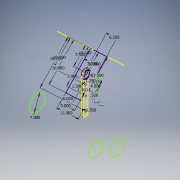
# Autodesk Inventor part: RollerIntakePrototype 2.0 3 WHEELS
Saved by Autodesk Inventor 2018.3 (Build 223284000, 284)
## iProperties
Created: 2020-01-29
Part Number: RollerIntakePrototype 2.0 3 WHEELS
Material: Generic
Document SubType Name: Modeling
Designer: 22oktynich
Density: 1 g/cm^3
Appearance: Default
Author: 22oktynich
Autodesk Inventor part; units mm, degrees
ref_plane "YZ Plane" through (0, 0, 0) normal (1, 0, 0) x (0, 1, 0)
ref_plane "XZ Plane" through (0, 0, 0) normal (0, 1, 0) x (-1, 0, 0)
ref_plane "XY Plane" through (0, 0, 0) normal (0, 0, 1) x (1, 0, 0)
sketch "Sketch1" plane through (0, 0, 0) normal (0, 0, 1) x (1, 0, 0)
  line L0 (0, 0) -> (-254, 0)
  line L1 (-254, 406.4) -> (0, 406.4)
  line L2 (0, 406.4) -> (0, 0)
  line L3 (-254, 0) -> (-254, 155.9052)
  line L4 (-285.75, 187.6552) -> (-355.6, 187.6552)
  circle A0 centre (-95.25, 190.5) radius 38.1
  arc A1 (-254, 155.9052) -> (-285.75, 187.6552) centre (-285.75, 155.9052) ccw
  circle A2 centre (-330.2, 463.55) radius 19.05
  line L5 (-515.6961, 0) -> (516.0768, 0) projected
  line L6 (-368.3, 304.8) -> (-355.6, 187.6552)
  circle A3 centre (-228.6, 355.6) radius 19.05
  circle A4 centre (279.7806, 579.9282) radius 88.9
  circle A5 centre (-152.4, 276.86) radius 19.05
  line L7 (-336.55, 187.6552) -> (-368.3, 304.8)
  point P0 (-254, 187.6552)
  dimension "d0" = 406.4
  dimension "d4" = 158.75
  dimension "d5" = 190.5
  dimension "d6" = 76.2
  dimension "d13" = 31.75
  dimension "d14" = 463.55
  dimension "d20" = 330.2
  dimension "d54" = 101.6
  dimension "d59" = 254
  dimension "d61" = 304.8
  dimension "d62" = 187.6552
  dimension "d63" = 12.7
  dimension "d76" = 38.1
  dimension "d87" = 228.6
  dimension "d88" = 355.6
  dimension "d89" = 38.1
  dimension "d90" = 177.8
  dimension "d91" = 38.1
  dimension "d92" = 276.86
  dimension "d93" = 152.4
  dimension "d94" = 82.55
  constraints: 14 end point, 6 centre point, 4 point on line, 2 point on circle, 2 tangent, 1 horizontal, 1 parallel, 1 vertical
  measures "d0" distance between parallel lines of L1 L0
  measures "d4" distance from line of L3 A0.centre
  measures "d5" distance from line of L0 A0.centre
  measures "d6" diameter of A0
  measures "d13" radius of A1
  measures "d14" distance from line of L0 A2.centre
  measures "d20" distance from line of L2 A2.centre
  measures "d54" distance from line of L4.end L3
  measures "d59" distance between parallel lines of L3 L2
  measures "d61" distance from line of L5 L6.start
  measures "d62" distance from line of L5 L4.end
  measures "d63" horizontal distance of L6.start L4.end
  measures "d76" diameter of A3
  measures "d87" distance from line of L2 A3.centre
  measures "d88" distance from line of L0 A3.centre
  measures "d89" diameter of A2
  measures "d90" diameter of A4
  measures "d91" diameter of A5
  measures "d92" distance from line of L5 A5.centre
  measures "d93" distance from line of L2 A5.centre
  measures "d94" distance from line of L3 L7.start
sketch "Sketch5" plane through (0, 0, 0) normal (0, 0, 1) x (1, 0, 0)
  line L0 (-346.559, 517.9919) -> (-91.3724, 246.8562)
  line L1 (-91.3724, 246.8562) -> (-49.3064, 146.7099)
  line L2 (-49.3064, 146.7099) -> (-96.1423, 127.0367)
  line L3 (-96.1423, 127.0367) -> (-134.6544, 218.7223)
  line L4 (-134.6544, 218.7223) -> (-383.5128, 483.1343)
  line L5 (-383.5128, 483.1343) -> (-346.5202, 517.9508)
  point P0 (0, 0)
  point P1 (-95.25, 190.5)
  point P2 (-152.4, 276.86)
  point P3 (-228.6, 355.6)
  point P4 (-330.2, 463.55)
  dimension "d107" = 50.8
  dimension "d108" = 50.8
  dimension "d109" = 25.4
  dimension "d110" = 25.4
  dimension "d111" = 25.4
  dimension "d113" = 50.8
  constraints: 12 end point, 3 perpendicular, 1 parallel, 1 point on line
  measures "d107" distance of L4.end L5.end
  measures "d108" distance from line of point (-330.2, 463.55) L5
  measures "d109" distance from line of L0 point (-330.2, 463.55)
  measures "d110" distance from line of L0 point (-228.6, 355.6)
  measures "d111" distance from line of L1 point (-95.25, 190.5)
  measures "d113" distance of L1.end L2.end
extrude "Extrusion4" add sketch "Sketch5" along normal blind 25.4
hole "Hole1" at (-95.25, 190.5, 0) at (-152.4, 276.86, 0) at (-228.6, 355.6, 0) at (-330.2, 463.55, 0) direction (0, 0, 1) diameter 22.225 end through all
sketch "Sketch6" plane through (0, 0, 25.4) normal (0, 0, 1) x (1, 0, 0)
  line L0 (-108.2166, 155.7818) -> (-61.3806, 175.455)
  line L1 (-49.3064, 146.7099) -> (-91.3724, 246.8562) projected
  line L2 (-61.3806, 175.455) -> (-49.3064, 146.7099)
  line L3 (-134.6544, 218.7223) -> (-96.1423, 127.0367) projected
  line L4 (-49.3064, 146.7099) -> (-96.1423, 127.0367)
  line L5 (-96.1423, 127.0367) -> (-108.2166, 155.7818)
  circle A0 centre (-95.25, 190.5) radius 11.1125 projected
  point P0 (0, 0)
  dimension "d123" = 26.9875
  constraints: 8 end point, 2 perpendicular, 2 point on line
  measures "d123" distance from line of A0.centre L0
extrude "Extrusion5" cut sketch "Sketch6" against normal blind 25.4 contours L0 L1 L4 L3
shell "Shell1" thickness 1.5875 removed faces 2 at (-92.6046, 162.3395, 8.4667) at (-358.8511, 506.3453, 8.4667)
sketch "Sketch7" plane through (-383.5128, 483.1343, 25.4) normal (-0.6854, 0.7282, 0) x (0.7282, 0.6854, 0)
  line L0 (49.2125, 1.5875) -> (1.5875, 1.5875) projected
  line L1 (1.5875, 1.5875) -> (1.5875, 23.8125) projected
  line L2 (49.2125, 1.5875) -> (1.5875, 1.5875)
  line L3 (1.5875, 1.5875) -> (1.5875, 23.8125)
  line L4 (1.5875, 23.8125) -> (49.2125, 23.8125)
  line L5 (49.2125, 23.8125) -> (49.2125, 1.5875)
  point P0 (-51.8492, 25.4)
  constraints: 8 end point, 2 parallel, 1 horizontal, 1 perpendicular
extrude "Extrusion6" cut sketch "Sketch7" against normal blind 330.2
sketch "Sketch8" plane through (-108.2166, 155.7818, 0) normal (0.3873, -0.922, 0) x (0.922, 0.3873, 0)
  line L0 (49.2125, 1.5875) -> (49.2125, 23.8125) projected
  line L1 (49.2125, 1.5875) -> (1.5875, 1.5875)
  line L2 (1.5875, 1.5875) -> (1.5875, 23.8125)
  line L3 (1.5875, 23.8125) -> (49.2125, 23.8125)
  line L4 (49.2125, 23.8125) -> (49.2125, 1.5875)
  point P0 (39.4428, 0)
  constraints: 8 end point, 2 parallel, 1 horizontal, 1 perpendicular
extrude "Extrusion7" cut sketch "Sketch8" against normal blind 76.2
sketch "Sketch9" plane through (0, 0, 25.4) normal (0, 0, 1) x (1, 0, 0)
  line L0 (-382.3568, 484.2223) -> (-133.3019, 219.6015) projected
  line L1 (-91.3724, 246.8562) -> (-346.5202, 517.9508) projected
  line L2 (-61.3806, 175.455) -> (-91.3724, 246.8562) projected
  line L3 (-91.3724, 246.8562) -> (-61.3806, 175.455)
  line L4 (-134.6544, 218.7223) -> (-108.2166, 155.7818) projected
  line L5 (-61.3806, 175.455) -> (-108.2166, 155.7818)
  line L6 (-108.2166, 155.7818) -> (-134.6544, 218.7223)
  line L7 (-383.5128, 483.1343) -> (-134.6544, 218.7223) projected
  line L8 (-91.3724, 246.8562) -> (-134.6544, 218.7223)
  line L9 (-91.3724, 246.8562) -> (-141.3682, 225.8557)
  line L10 (-91.3724, 246.8562) -> (-130.8608, 209.6907)
  line L11 (-346.5202, 517.9508) -> (-383.5128, 483.1343) projected
  point P0 (0, 0)
  constraints: 12 end point, 2 collinear, 2 parallel, 2 point on line, 1 perpendicular
sketch "Sketch10" plane through (0, 0, 25.4) normal (0, 0, 1) x (1, 0, 0)
  circle A0 centre (-948.4671, 602.0735) radius 85.2109
  circle A1 centre (-704.3018, 697.4759) radius 79.8897
  point P0 (0, 0)
  constraints: 2 centre point
sketch "Sketch11" plane through (0, 0, 0) normal (0, 0, -1) x (-1, 0, 0)
  line L0 (61.3806, 175.455) -> (91.3724, 246.8562) projected
  line L1 (91.3724, 246.8562) -> (141.3682, 225.8557)
  line L2 (383.5128, 483.1343) -> (134.6544, 218.7223) projected
  line L3 (61.3806, 175.455) -> (108.2166, 155.7818) projected
  line L4 (134.6544, 218.7223) -> (108.2166, 155.7818) projected
  line L5 (91.3724, 246.8562) -> (134.6544, 218.7223)
  line L6 (91.3724, 246.8562) -> (346.5202, 517.9508) projected
  line L7 (91.3724, 246.8562) -> (130.8607, 209.6906)
  point P0 (0, 0)
  dimension "d131" = 10.24
  constraints: 6 end point, 2 point on line, 1 parallel
  measures "d131" angle of L7 L5
body "Solid4"
